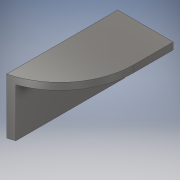
# Autodesk Inventor part: RearWheelMount
Saved by Autodesk Inventor 2017 (Build 210142000, 142)
## iProperties
Created: 2017-01-30
Part Number: RearWheelMount
Material: Steel, Mild
Document SubType Name: Sheet Metal
Designer: Robert.Chapman
Density: 7.85 g/cm^3
Sheet Metal Rule: Default
Appearance: Semi-Polished
Mass: 203.51 g
Surface Area: 122.933 cm^2
Volume: 25.9248 cm^3
Author: Robert.Chapman
Autodesk Inventor part; units mm, degrees
ref_plane "YZ Plane" through (0, 0, 0) normal (1, 0, 0) x (0, 1, 0)
ref_plane "XZ Plane" through (0, 0, 0) normal (0, 1, 0) x (-1, 0, 0)
ref_plane "XY Plane" through (0, 0, 0) normal (0, 0, 1) x (1, 0, 0)
sketch "Sketch1" plane through (0, 0, 0) normal (0, 0, 1) x (1, 0, 0)
  line L0 (0, 12.6249) -> (38.1, 12.6249)
  line L1 (38.1, 12.6249) -> (38.1, 7.8624)
  line L2 (38.1, 7.8624) -> (4.7625, 7.8624)
  line L3 (4.7625, 7.8624) -> (4.7625, -25.4751)
  line L4 (4.7625, -25.4751) -> (0, -25.4751)
  line L5 (0, -25.4751) -> (0, 12.6249)
  point P0 (0, 0)
  dimension "d0" = 38.1
  dimension "d1" = 4.7625
  dimension "d2" = 4.7625
  dimension "d3" = 38.1
  constraints: 12 end point, 5 perpendicular, 1 horizontal
  measures "d0" distance of L0.start L0.end
  measures "d1" distance of L0.end L1.end
  measures "d2" distance of L3.end L4.end
  measures "d3" distance of L4.end L0.start
extrude "Extrusion1" add sketch "Sketch1" along normal blind 76.2
fillet "Corner Round2" radius 50.8 1 edges at (38.1, 10.2436, 76.2)
equation "\"BendRadius\" = Thickness"
equation "\"BendReliefWidth\" = Thickness"
equation "\"BendReliefDepth\" = 0.5 * Thickness"
equation "\"CornerReliefSize\" = 4 * Thickness"
equation "\"MinimumRemnant\" = 2 * Thickness"
equation "\"TransitionRadius\" = BendRadius"
equation "\"JacobiRadiusSize\" = BendRadius"
equation "\"GapSize\" = Thickness"
equation "\"Thickness\" = 4.7625"
body "Solid1"
